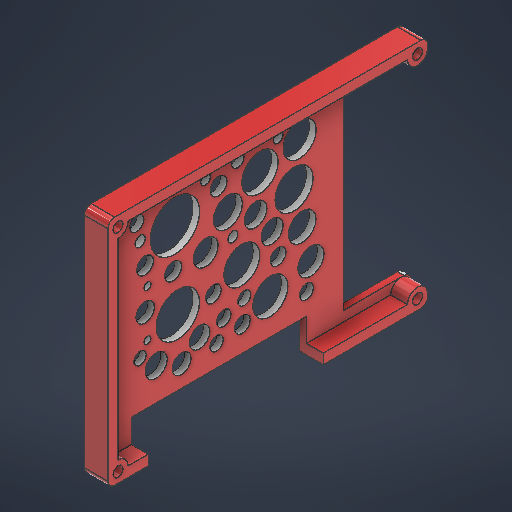
# Autodesk Inventor part: RP5_cover
Saved by Autodesk Inventor 2026.1 (Build 301233000, 233)
## iProperties
Created: 2025-12-08
Part Number: RP5_cover
Material: Generic
Document SubType Name: Modeling
Designer: emanuel
Density: 1 g/cm^3
Appearance: Default
Author: emanuel
Autodesk Inventor part; units mm, degrees
ref_plane "YZ Plane" through (0, 0, 0) normal (1, 0, 0) x (0, 1, 0)
ref_plane "XZ Plane" through (0, 0, 0) normal (0, 1, 0) x (-1, 0, 0)
ref_plane "XY Plane" through (0, 0, 0) normal (0, 0, 1) x (1, 0, 0)
sketch "Sketch1" plane through (0, 0, 0) normal (1, 0, 0) x (0, 1, 0)
  line L0 (0, 0) -> (69, 0)
  line L1 (69, 0) -> (69, -95)
  line L2 (69, -95) -> (0, -95)
  line L3 (0, -95) -> (0, 0)
  line L4 (69, 0) -> (66, 0)
  line L5 (66, 0) -> (66, -3)
  line L6 (66, -3) -> (69, -3)
  line L7 (69, -3) -> (69, 0)
  line L8 (0, -95) -> (3, -95)
  line L9 (3, -95) -> (3, -92)
  line L10 (3, -92) -> (0, -92)
  line L11 (0, -92) -> (0, -95)
  circle A0 centre (66, -3) radius 1.5
  circle A1 centre (3, -92) radius 1.5
  circle A2 centre (66, -92) radius 1.5
  circle A3 centre (3, -3) radius 1.5
  line L12 (34.5, 0) -> (34.5, -95)
  line L13 (69, 0) -> (34.5, 0)
  line L14 (51.75, 0) -> (51.75, -95)
  line L15 (34.5, -95) -> (0, -95)
  line L16 (17.25, -95) -> (17.25, 0)
  line L17 (69, 0) -> (69, -17.5)
  line L18 (69, -17.5) -> (69, -37.5)
  line L19 (69, -37.5) -> (69, -57.5)
  line L20 (69, -57.5) -> (69, -77.5)
  line L21 (69, -17.5) -> (0, -17.5)
  line L22 (69, -37.5) -> (0, -37.5)
  line L23 (69, -57.5) -> (0, -57.5)
  line L24 (69, -77.5) -> (0, -77.5)
  circle A4 centre (51.75, -17.5) radius 7.5
  circle A5 centre (51.75, -37.5) radius 7.5
  circle A6 centre (51.75, -57.5) radius 7.5
  circle A7 centre (51.75, -77.5) radius 7.5
  circle A8 centre (34.5, -17.5) radius 7.5
  circle A9 centre (34.5, -37.5) radius 7.5
  circle A10 centre (34.5, -57.5) radius 7.5
  circle A11 centre (34.5, -77.5) radius 7.5
  circle A12 centre (17.25, -17.5) radius 7.5
  circle A13 centre (17.25, -37.5) radius 7.5
  circle A14 centre (17.25, -57.5) radius 7.5
  circle A15 centre (17.25, -77.5) radius 7.5
  circle A16 centre (51.75, -17.5) radius 17.25
  circle A17 centre (51.75, -37.5) radius 17.25
  circle A18 centre (51.75, -57.5) radius 17.25
  circle A19 centre (51.75, -77.5) radius 17.25
  circle A20 centre (34.5, -17.5) radius 17.25
  circle A21 centre (34.5, -37.5) radius 17.25
  circle A22 centre (34.5, -57.5) radius 17.25
  circle A23 centre (34.5, -77.5) radius 17.25
  circle A24 centre (17.25, -17.5) radius 17.25
  circle A25 centre (17.25, -37.5) radius 17.25
  circle A26 centre (17.25, -57.5) radius 17.25
  circle A27 centre (17.25, -77.5) radius 17.25
  line L25 (0, 0) -> (0, -12)
  line L26 (0, -12) -> (10, -12)
  line L27 (10, -12) -> (10, -64)
  line L28 (10, -64) -> (0, -64)
  line L29 (0, -64) -> (0, -12)
  point P0 (42, -17.5)
  point P1 (36.1304, -10.1794)
  point P2 (43.125, -2.5611)
  point P3 (50.1196, -10.1794)
  point P4 (59.25, -17.5)
  point P5 (51.75, -20.25)
  point P6 (65.8057, -27.5)
  point P7 (58.1149, -33.5328)
  point P8 (51.75, -30)
  point P9 (51.75, -25)
  point P10 (45.3851, -21.4672)
  point P11 (51.5292, -20.2514)
  point P12 (34.5, -17.5)
  point P13 (36.1304, -24.8206)
  point P14 (40.8649, -21.4672)
  point P15 (48.5557, -27.5)
  point P16 (20.4443, -27.5)
  point P17 (28.1351, -21.4672)
  point P18 (32.8696, -24.8206)
  point P19 (58.1149, -61.4672)
  point P20 (65.8057, -67.5)
  point P21 (51.75, -74.75)
  point P22 (59.25, -77.5)
  point P23 (50.1196, -84.8206)
  point P24 (43.125, -92.4389)
  point P25 (36.1304, -84.8206)
  point P26 (42, -77.5)
  point P27 (51.5292, -74.7486)
  point P28 (45.3851, -73.5328)
  point P29 (51.75, -70)
  point P30 (51.75, -65)
  point P31 (48.5557, -47.5)
  point P32 (20.4443, -47.5)
  point P33 (34.5, -77.5)
  point P34 (32.8696, -70.1794)
  point P35 (28.1351, -73.5328)
  point P36 (25.875, -72.4389)
  point P37 (17.4708, -74.7486)
  point P38 (27, -77.5)
  point P39 (32.8696, -84.8206)
  point P40 (25.875, -92.4389)
  point P41 (18.8804, -84.8206)
  point P42 (9.75, -77.5)
  point P43 (17.25, -74.75)
  point P44 (3.1943, -67.5)
  point P45 (10.8851, -61.4672)
  point P46 (17.25, -65)
  point P47 (17.25, -70)
  point P48 (18.8804, -70.1794)
  point P49 (48.5557, -67.5)
  point P50 (40.8649, -73.5328)
  point P51 (36.1304, -70.1794)
  point P52 (25.875, -2.5611)
  point P53 (32.8696, -10.1794)
  point P54 (27, -17.5)
  point P55 (17.4708, -20.2514)
  point P56 (23.6149, -21.4672)
  point P57 (17.25, -25)
  point P58 (17.25, -30)
  point P59 (10.8851, -33.5328)
  point P60 (3.1943, -27.5)
  point P61 (17.25, -20.25)
  point P62 (9.75, -17.5)
  point P63 (18.8804, -10.1794)
  point P64 (23.6149, -73.5328)
  point P65 (20.4443, -67.5)
  point P66 (17.25, -60.25)
  point P67 (17.25, -50)
  point P68 (17.25, -45)
  point P69 (10, -17.5)
  point P70 (10, -19.4203)
  point P71 (10, -57.5)
  point P72 (18.8804, -24.8206)
  point P73 (10.8851, -73.5328)
  point P74 (58.1149, -73.5328)
  dimension "d0" = 69
  dimension "d1" = 95
  dimension "d2" = 3
  dimension "d3" = 3
  dimension "d4" = 3
  dimension "d5" = 3
  dimension "d6" = 3
  dimension "d7" = 3
  dimension "d8" = 3
  dimension "d9" = 3
  dimension "d10" = 17.5
  dimension "d11" = 20
  dimension "d12" = 20
  dimension "d13" = 20
  dimension "d14" = 15
  dimension "d15" = 15
  dimension "d16" = 15
  dimension "d17" = 15
  dimension "d18" = 15
  dimension "d19" = 15
  dimension "d20" = 15
  dimension "d21" = 15
  dimension "d22" = 15
  dimension "d23" = 15
  dimension "d24" = 15
  dimension "d25" = 15
  dimension "d40" = 12
  dimension "d41" = 10
  dimension "d42" = 52
  constraints: 60 end point, 19 point on line, 16 centre point, 14 coincident, 10 perpendicular, 8 parallel, 4 horizontal, 4 midpoint, 2 collinear, 36 other
  measures "d0" distance of L1.end L2.end
  measures "d1" distance of L0.end L1.end
  measures "d2" distance of L6.end L5.end
  measures "d3" distance of L5.end L4.end
  measures "d4" distance of L10.end L9.end
  measures "d5" distance of L9.end L8.end
  measures "d6" diameter of A0
  measures "d7" diameter of A1
  measures "d8" diameter of A2
  measures "d9" diameter of A3
  measures "d10" distance of L0.end L17.end
  measures "d11" distance of L17.end L18.end
  measures "d12" distance of L18.end L19.end
  measures "d13" distance of L19.end L20.end
  measures "d14" diameter of A4
  measures "d15" diameter of A5
  measures "d16" diameter of A6
  measures "d17" diameter of A7
  measures "d18" diameter of A8
  measures "d19" diameter of A9
  measures "d20" diameter of A10
  measures "d21" diameter of A11
  measures "d22" diameter of A12
  measures "d23" diameter of A13
  measures "d24" diameter of A14
  measures "d25" diameter of A15
  measures "d40" distance of L0.start L25.end
  measures "d41" distance of L27.end L28.end
  measures "d42" distance of L26.end L27.end
extrude "Extrusion1" add sketch "Sketch1" along normal blind 2 contours L0 L16 A24 L26 L3 | L0 L12 A20 A24 L16 | L0 L14 A16 A20 L12 | A24 A20 A12 L16 | L16 A12 L27 L26 A24 | L0 L5 A0 L6 L1 A16 L14 | A20 A16 A8 L12 | L12 A8 A24 A20 | A12 A20 L16 | L16 L21 L27 A12 | A24 A8 L21 A12 A20 | L21 L27 A12 | L0 L1 L6 A0 L5 | A16 L21 A4 L14 | L14 A4 A20 A16 | A8 A16 L12 | L12 A24 A8 | A20 A4 L21 A8 A16 | A20 A25 L16 | A20 A12 L21 | L16 A25 A12 L27 L21 | L21 A12 A25 A20 | A24 L21 A8 | A12 A25 L27 | L27 A25 A12 L16 A13 A24 | A24 A13 L27 | A4 L21 L14 | L14 A20 A4 | A16 A17 A4 L21 | L1 A17 A16 | A16 A21 L12 | A16 A8 L21 | A24 A21 A8 L21 | L21 A8 A21 A16 | L12 A21 A24 | A20 L21 A4 | A25 A20 A12 L16 | L16 A12 A25 | L21 A8 A21 A25 A12 | A25 A12 A20 | L28 A26 A27 L3 | L28 A27 A26 | L27 A13 A24 L16 L22 | L22 L16 A26 A13 L27 | A13 A26 L27 | L27 A26 A13 L16 A14 A25 | A25 A14 L27 | A13 L16 A24 | L21 A4 A17 L14 | A20 A17 A4 L21 | L14 A17 A20 | A17 A18 A5 L22 | L22 A5 A16 A17 | L1 A18 A17 | A16 A5 L14 A4 A17 | A21 A16 A8 L12 | L12 A8 A24 A21 | L21 A4 A17 A21 A8 | A21 A8 A16 | A24 A8 A21 | A12 A20 A21 A13 L16 | A25 A21 A20 A12 | A8 A24 A25 A21 | A27 L16 L2 L9 A1 L10 L3 | A27 A26 A15 L24 | L24 A15 L16 A27 | L27 A14 A25 L16 L23 | L23 L16 A27 A14 L27 | A14 A27 L27 | A27 L28 L27 A14 L16 A15 A26 | A21 A26 L16 | A21 A24 A13 L22 | L16 A24 A21 | L22 A13 A26 A21 | A26 L16 A13 | A14 L16 A25 | A13 A21 A24 L16 | A17 A4 L14 | L14 A4 A20 A17 | A20 A4 A17 | A18 A19 A6 L23 | L23 A6 A17 A18 | L1 A19 A18 | A5 A18 L14 L22 | L22 L14 A16 A5 | A17 A6 L14 A5 A18 | A16 L14 A5 | A8 A16 A17 A9 L12 | L12 A9 A25 A24 A8 | A21 A17 A16 A8 | A4 A20 A21 A17 | A25 A24 A20 A21 | A20 A24 A13 A21 | L10 A1 L9 L2 L3 | A15 A26 L16 L24 | L24 L16 A15 | A27 A23 L12 L2 L16 | L16 A15 A23 A27 | A22 A27 L16 | A22 A25 A14 L23 | L16 A25 A22 | L23 A14 A27 A22 | A27 L16 A14 | A15 L16 A26 | A26 A21 A13 L16 | A13 A24 A20 A9 L22 | L22 A9 A22 A26 A13 | A21 A13 A24 | A26 A13 A21 | A13 A21 A22 A14 L16 | A14 A22 A25 L16 | L14 A5 A21 A20 A4 | A19 L14 A7 L24 | L24 A7 A18 A19 | L1 L2 L14 A19 | A6 A19 L14 L23 | L23 L14 A17 A6 | A18 A7 L14 A6 A19 | A21 A16 L14 | A21 A18 A5 L22 | L22 A5 A16 A21 | L14 A18 A21 | A5 L14 A18 | A17 L14 A6 | L14 A16 A21 A5 | A9 A17 A20 L12 | L12 A20 A25 A9 | A21 A20 A16 A17 | A16 A20 A9 A17 | A25 A9 A20 A24 | A23 A15 L16 | A23 A26 A15 L24 | L16 A26 A23 | L24 A15 A23 | A27 A11 L12 A23 | A23 A15 L24 A11 A27 | A27 A22 A14 L16 | A14 A25 A21 A10 L23 | L23 A10 A23 A27 A14 | A22 A14 A25 | A27 A14 A22 | A14 A22 A23 A15 L16 | A15 A23 A26 L16 | A9 A20 A25 L22 | L22 A25 A22 A9 | A26 A22 A21 A13 | A22 A21 A25 A14 | A21 A5 A16 A20 | A7 L14 L24 | L24 L14 A18 A7 | A19 A23 A7 L14 | L14 L2 L12 A23 A19 | A22 A17 L14 | A22 A19 A6 L23 | L23 A6 A17 A22 | L14 A19 A22 | A6 L14 A19 | A18 L14 A7 | L14 A5 A21 A18 | A5 A18 A22 A9 L22 | L22 A9 A20 A16 A5 | A16 A5 A21 | A21 A5 A18 | L14 A6 A22 A21 A5 | L14 A17 A22 A6 | A20 A17 L12 | L12 A25 A20 | A9 A20 A17 | A25 A20 A9 | A15 A26 A22 A11 L24 | A23 A15 A26 | L12 A11 A19 A23 | A27 L12 A11 | A11 L24 A27 | A10 A21 A26 L23 | L23 A26 A23 A10 | A27 A23 A22 A14 | A23 A22 A26 A15 | A17 A22 L12 | A17 A20 A9 L22 | L22 A9 A22 A17 | L12 A22 A25 | A22 A25 A9 | A9 A25 A26 A22 | A26 A25 A21 A22 | A23 A18 L14 | A23 A7 L24 | L24 A7 A18 A23 | L14 A7 A23 | A19 A11 L24 A7 A23 | L14 A6 A22 A19 | A6 A19 A23 A10 L23 | L23 A10 A21 A17 A6 | A17 A6 A22 | A22 A6 A19 | L14 A7 A23 A22 A6 | L14 A18 A23 A7 | A5 A21 A22 A18 | A6 A17 A21 A22 | A11 A22 A27 L24 | L12 A19 A11 | A27 A22 L12 | A19 A22 A11 L24 | L12 A22 A19 | L24 A11 A19 | A26 A21 L12 | A18 A23 L12 | A18 A21 A10 L23 | L12 A21 A18 | L23 A10 A23 A18 | L12 A23 A26 | A21 A25 A26 A10 | A10 A26 A21 | A23 A26 A10 | A10 A26 A27 A23 | A27 A26 A22 A23 | A22 A17 A9 L12 | L12 A9 A25 A22 | A22 A9 A17 | A9 L12 A10 A26 A25 | L24 A11 A22 A18 A7 | A18 A7 A23 | A6 A22 A23 A19 | A7 A18 A22 A23 | A22 A18 A17 A9 | A22 A21 A17 A18 | A22 A26 A27 A11 | A11 A27 A22 | A22 A27 A11 L12 | L12 A11 A19 A22 | A19 A11 A22 | A21 A26 A10 L12 | L12 A10 A18 A21 | A23 A18 A10 L12 | L12 A10 A26 A23 | A18 A10 A21 | A23 A10 A18 | A10 L12 A11 A27 A26 | A9 A17 A18 A10 L12 | A10 A18 A17 A21 | A23 A19 A18 A10 | A23 A22 A18 A19 | L12 A10 A18 A19 A11 | A11 A19 A18 A22 picked at (9.9538, -18.5695)
sketch "Sketch2" plane through (2, 0, 0) normal (1, 0, 0) x (0, 0, -1)
  line L0 (95, 69) -> (0, 69) projected
  line L1 (0, 0) -> (95, 0) projected
  line L2 (0, 69) -> (3, 69)
  line L3 (3, 69) -> (3, 0)
  line L4 (3, 0) -> (0, 0)
  line L5 (0, 0) -> (0, 69)
  line L6 (95, 0) -> (95, 69) projected
  line L7 (0, 69) -> (95, 69)
  line L8 (95, 69) -> (95, 66)
  line L9 (95, 66) -> (0, 66)
  line L10 (0, 66) -> (0, 69)
  line L11 (0, 0) -> (95, 0)
  line L12 (95, 0) -> (95, 3)
  line L13 (95, 3) -> (0, 3)
  line L14 (0, 3) -> (0, 0)
  circle A0 centre (3, 66) radius 1.5 projected
  circle A1 centre (3, 66) radius 3
  circle A2 centre (92, 66) radius 1.5 projected
  circle A3 centre (92, 66) radius 3
  circle A4 centre (92, 3) radius 1.5 projected
  circle A5 centre (92, 3) radius 3
  circle A6 centre (3, 3) radius 1.5 projected
  circle A7 centre (3, 3) radius 3
  point P0 (89, 3)
  point P1 (6, 3)
  point P2 (3, 6)
  point P3 (3, 63)
  point P4 (6, 66)
  point P5 (89, 66)
  dimension "d29" = 3
  dimension "d30" = 3
  dimension "d31" = 3
  constraints: 24 end point, 6 parallel, 4 coincident, 3 horizontal, 3 perpendicular, 3 point on line, 2 centre point, 2 tangent, 6 other
  measures "d29" distance of L3.end L4.end
  measures "d30" distance of L7.end L8.end
  measures "d31" distance of L12.end L11.end
extrude "Extrusion2" add sketch "Sketch2" along normal blind 5 contours A1 L5 L0 | A1 L9 A0 L3 | L0 A3 L9 A1 | L3 A0 L9 A1 | L0 L6 A3 | A3 L9 A2 | A1 L3 A0 L9 | A1 L3 A7 L5 | L9 A0 L3 A1 | A3 L9 A2 | A7 L1 L5 | A7 L3 A6 L13 | L13 A6 L3 A7 | A5 L13 A4 | L13 A4 A5 | L6 L1 A5 | A7 L13 A6 L3 | A7 L13 A5 L1 | L3 A6 L13 A7
fillet "Fillet2" radius 2 4 edges at (3.5, 0, 0) (3.5, 69, 0) (3.5, 69, -95) (3.5, 0, -95)
sketch "Sketch3" plane through (0, 0, -93) normal (0, -1, 0) x (1, 0, 0)
  line L0 (0, 93) -> (0, 81)
  line L1 (0, 81) -> (0, 29)
  line L2 (0, 29) -> (10, 29)
  line L3 (10, 29) -> (10, 81)
  line L4 (10, 81) -> (0, 81)
  line L5 (0, 81) -> (0, 29)
  dimension "d35" = 12
  dimension "d36" = 52
  dimension "d37" = 10
  constraints: 12 end point, 2 parallel, 1 horizontal, 1 perpendicular, 1 point on line, 1 vertical
  measures "d35" distance of L0.start L0.end
  measures "d36" distance of L0.end L1.end
  measures "d37" distance of L4.end L3.end
extrude "Extrusion3" cut sketch "Sketch3" against normal blind 10
sketch "Sketch5" plane through (2, 0, 0) normal (1, 0, 0) x (0, 0, -1)
  line L0 (77.5, 42) -> (77.5, 59.25) projected
  line L1 (95, 3) -> (95, 66) projected
  line L2 (77.5, 59.25) -> (95, 59.25)
  line L3 (95, 59.25) -> (95, 63)
  line L4 (95, 63) -> (77.5, 63)
  line L5 (77.5, 63) -> (77.5, 59.25)
  line L6 (77.5, 9.75) -> (95, 9.75)
  line L7 (95, 9.75) -> (95, 6)
  line L8 (95, 6) -> (77.5, 6)
  line L9 (77.5, 6) -> (77.5, 9.75)
  line L10 (95, 6) -> (75, 6)
  line L11 (75, 6) -> (75, 59.25)
  line L12 (75, 59.25) -> (95, 59.25)
  line L13 (95, 59.25) -> (95, 6)
  line L14 (77.5, 59.25) -> (75, 59.25)
  line L15 (75, 59.25) -> (75, 63)
  line L16 (75, 63) -> (77.5, 63)
  line L17 (77.5, 63) -> (77.5, 59.25)
  point P0 (0, 0)
  dimension "d55" = 3.75
  dimension "d56" = 3.75
  dimension "d57" = 20
  constraints: 32 end point, 8 parallel, 4 horizontal, 4 perpendicular, 3 point on line
  measures "d55" distance of L3.end L2.end
  measures "d56" distance of L6.end L7.end
  measures "d57" distance of L11.end L12.end
extrude "Extrusion6" cut sketch "Sketch5" against normal blind 5
fillet "Fillet5" radius 2 2 edges at (1, 63, -95) (1, 6, -95)
sketch "Sketch6" plane through (0, 0, 0) normal (-1, 0, 0) x (0, 0, 1)
  line L0 (-75, 63) -> (-70, 63)
  line L1 (-70, 63) -> (-10, 63)
  line L2 (-10, 63) -> (-10, 13)
  line L3 (-10, 13) -> (-70, 13)
  line L4 (-70, 13) -> (-70, 63)
  circle A0 centre (-61.9538, 56.5437) radius 4.9265
  circle A1 centre (-50.1881, 53.9291) radius 5.4099
  circle A2 centre (-60.3197, 44.5601) radius 5.6618
  circle A3 centre (-48.8808, 43.6886) radius 3.356
  circle A4 centre (-53.7831, 36.9342) radius 3.2683
  circle A5 centre (-62.7164, 33.6659) radius 4.1009
  circle A6 centre (-55.598, 29.565) radius 2.3267
  circle A7 centre (-44.7782, 32.7944) radius 5.3456
  circle A8 centre (-42.1264, 41.4008) radius 1.4818
  circle A9 centre (-40.6446, 48.5192) radius 4.3155
  circle A10 centre (-37.8777, 56.5437) radius 2.5026
  circle A11 centre (-43.6082, 60.2477) radius 1.852
  circle A12 centre (-25.7851, 29.565) radius 6.432
  circle A13 centre (-53.2713, 20.484) radius 5.2109
  circle A14 centre (-24.9136, 52.8346) radius 7.3452
  circle A15 centre (-34.0647, 41.4008) radius 3.6746
  circle A16 centre (-39.4326, 21.7913) radius 2.1393
  circle A17 centre (-19.3531, 19.652) radius 3.2886
  circle A18 centre (-16.0645, 34.9732) radius 2.753
  circle A19 centre (-24.3689, 41.4008) radius 2.5249
  circle A20 centre (-16.0645, 47.0446) radius 2.4778
  circle A21 centre (-13.5867, 59.0463) radius 2.0915
  circle A22 centre (-14.5641, 54.0411) radius 1.5527
  circle A23 centre (-16.743, 41.4008) radius 1.0649
  circle A24 centre (-16.743, 27.4488) radius 1.0649
  circle A25 centre (-14.5641, 23.9305) radius 1.8414
  circle A26 centre (-32.2588, 20.484) radius 3.0391
  circle A27 centre (-36.3292, 29.565) radius 2.3255
  circle A28 centre (-65.331, 23.5231) radius 3.8711
  circle A29 centre (-64.0237, 16.3634) radius 2.0699
  circle A30 centre (-44.9601, 17.4449) radius 2.3365
  circle A31 centre (-45.5247, 23.9305) radius 1.9261
  circle A32 centre (-37.2933, 16.3634) radius 1.9954
  circle A33 centre (-26.8938, 16.3634) radius 2.8112
  circle A34 centre (-34.0037, 60.1798) radius 1.4595
  circle A35 centre (-55.598, 60.1798) radius 1.4595
  point P0 (0, 0)
  dimension "d61" = 5
  dimension "d62" = 60
  dimension "d63" = 50
  constraints: 36 centre point, 10 end point, 2 horizontal, 2 parallel, 1 perpendicular
  measures "d61" distance of L0.start L0.end
  measures "d62" distance of L2.end L3.end
  measures "d63" distance of L1.end L2.end
extrude "Extrusion7" cut sketch "Sketch6" against normal blind 10 contours A0 | A1 | A2 | A3 | A4 | A5 | A6 | A7 | A8 | A9 | A10 | A11 | A12 | A13 | A14 | A15 | A16 | A17 | A18 | A19 | A20 | A21 | A22 | A23 | A24 | A25 | A26 | A27 | A28 | A29 | A30 | A31 | A32 | A33 | A34 | A35
body "Solid1"
